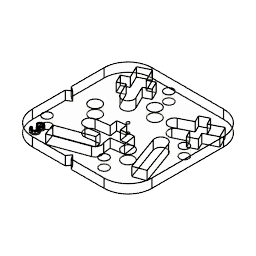
TopPlateTest_v2 (Autodesk Fusion 360 design; units mm, degrees)
Autodesk Fusion 360 part; units mm, degrees
sketch "Sketch1" plane through (0, 0, 0) normal (0, 0, 1) x (1, 0, 0)
  line L0 (55, -55) -> (-55, -55)
  line L1 (-55, -55) -> (-55, 55)
  line L2 (-55, 55) -> (55, 55)
  line L3 (55, 55) -> (55, -55)
  circle A0 centre (0, 9) radius 2
  circle A1 centre (0, -11) radius 1
  circle A2 centre (0, 0) radius 0.5
  circle A3 centre (-27, 47) radius 3
  circle A4 centre (-1, 47) radius 3
  circle A5 centre (46.8686, 27.2241) radius 3
  line L4 (46.9988, 1) -> (46.9855, 27.035) construction
  line L5 (-1, 47) -> (-27, 47) construction
  circle A6 centre (47.0008, 0.9939) radius 3
  circle A7 centre (-47, -1) radius 3
  line L6 (-47.008, -2.9175) -> (-47.0012, -29) construction
  circle A8 centre (-47, -27) radius 3
  circle A9 centre (0.0158, -47.1318) radius 3
  line L7 (1, -47) -> (27, -47) construction
  circle A10 centre (27.9746, -46.6245) radius 3
  line L8 (27.9746, -46.6245) -> (11, 0) construction
  line L9 (0, 0) -> (5, 0) construction
  line L10 (9.1207, -0.6842) -> (12.8793, 0.6842) construction
  line L11 (12.8793, 0.6842) -> (16.9846, -10.5917)
  line L12 (9.1207, -0.6842) -> (13.2259, -11.9602)
  line L13 (16.9846, -10.5917) -> (13.2259, -11.9602)
  circle A11 centre (11, 0) radius 2
  line L14 (-0.6842, -9.1207) -> (-11.9602, -13.2259)
  line L15 (-10.5917, -16.9846) -> (-11.9602, -13.2259)
  line L16 (0.6842, -12.8793) -> (-10.5917, -16.9846)
  circle A12 centre (0, -11) radius 2
  line L17 (-46.6245, -27.9746) -> (0, -11) construction
  circle A13 centre (7.7782, 7.7782) radius 2
  line L18 (7.7782, 7.7782) -> (46.8686, 27.2241) construction
  line L19 (7.7782, 7.7782) -> (8.669, 5.9875) construction
  line L20 (8.669, 5.9875) -> (19.413, 11.3322)
  line L21 (19.413, 11.3322) -> (17.6314, 14.9136)
  line L22 (17.6314, 14.9136) -> (6.8874, 9.5688)
  circle A14 centre (-7.7782, 7.7782) radius 2
  line L23 (-7.7782, 7.7782) -> (-27, 47) construction
  line L24 (-7.7782, 7.7782) -> (-9.5741, 6.898) construction
  line L25 (-9.5741, 6.898) -> (-14.855, 17.6736)
  line L26 (-5.9823, 8.6583) -> (-11.2631, 19.4339)
  line L27 (-11.2631, 19.4339) -> (-14.855, 17.6736)
  line L28 (46.9988, 1) -> (-6.364, -6.364) construction
  line L29 (0.0158, -47.1318) -> (-11, 0) construction
  line L30 (0, 9) -> (-47.008, -2.9175) construction
  circle A15 centre (7.7782, -7.7782) radius 2
  line L31 (7.7782, -7.7782) -> (-1, 47) construction
  line L32 (0, 0) -> (9, 0) construction
  circle A16 centre (-6.364, -6.364) radius 2
  line L33 (0, -11) -> (0.6842, -12.8793)
  circle A17 centre (-11, 0) radius 2
  line L34 (-11, 0) -> (-9.0525, 0.4552) construction
  line L35 (-9.0525, 0.4552) -> (-6.3214, -11.2299)
  line L36 (-6.3214, -11.2299) -> (-10.2164, -12.1403)
  line L37 (-10.2164, -12.1403) -> (-12.9475, -0.4552)
  line L38 (-6.364, -6.364) -> (-6.0906, -8.3452) construction
  line L39 (-6.0906, -8.3452) -> (5.7968, -6.7048)
  line L40 (5.7968, -6.7048) -> (5.25, -2.7423)
  line L41 (5.25, -2.7423) -> (-6.6374, -4.3827)
  line L42 (7.7782, -7.7782) -> (9.753, -7.4617) construction
  line L43 (9.753, -7.4617) -> (7.8542, 4.3871)
  line L44 (7.8542, 4.3871) -> (3.9046, 3.7542)
  line L45 (3.9046, 3.7542) -> (5.8034, -8.0946)
  line L46 (0, 9) -> (0.4915, 7.0613) construction
  line L47 (0.4915, 7.0613) -> (-11.1405, 4.1124)
  line L48 (-11.1405, 4.1124) -> (-12.1235, 7.9897)
  line L49 (-12.1235, 7.9897) -> (-0.4915, 10.9387)
  line L50 (20, -20) -> (-20, -20)
  line L51 (-20, -20) -> (-20, 20)
  line L52 (-20, 20) -> (20, 20)
  line L53 (20, 20) -> (20, -20)
  line L54 (20, -20) -> (-20, 20) construction
  line L55 (-20, -20) -> (20, 20) construction
  line L56 (15.1052, -11.276) -> (11, 0) construction
  line L57 (13.0526, -5.638) -> (14.9319, -4.9538) construction
  line L58 (13.0526, -5.638) -> (11.1733, -6.3222) construction
  line L59 (14.9319, -4.9538) -> (17.2811, -4.0985) construction
  line L60 (16.7679, -2.689) -> (17.7943, -5.508)
  line L61 (17.7943, -5.508) -> (9.3373, -8.5869)
  line L62 (16.7679, -2.689) -> (8.311, -5.7679)
  line L63 (8.311, -5.7679) -> (9.3373, -8.5869)
  line L64 (18.5222, 13.1229) -> (7.7782, 7.7782) construction
  line L65 (13.1502, 10.4505) -> (14.041, 8.6599) construction
  line L66 (14.041, 8.6599) -> (15.1545, 6.4215) construction
  line L67 (13.8115, 5.7534) -> (16.4975, 7.0896)
  line L68 (13.8115, 5.7534) -> (9.8029, 13.8115)
  line L69 (9.8029, 13.8115) -> (12.4889, 15.1476)
  line L70 (12.4889, 15.1476) -> (16.4975, 7.0896)
  line L71 (-13.0591, 18.5537) -> (-7.7782, 7.7782) construction
  line L72 (-10.4186, 13.1659) -> (-6.3778, 15.1463) construction
  line L73 (-7.0379, 16.4932) -> (-5.7177, 13.7993)
  line L74 (-7.0379, 16.4932) -> (-5.7177, 13.7993) construction
  line L75 (-5.7177, 13.7993) -> (-13.7993, 9.8387)
  line L76 (-13.7993, 9.8387) -> (-15.1196, 12.5326)
  line L77 (-15.1196, 12.5326) -> (-7.0379, 16.4932)
  line L78 (0, 9) -> (-11.632, 6.051) construction
  line L79 (-5.816, 7.5255) -> (-4.7101, 3.1635) construction
  line L80 (-6.1642, 2.7949) -> (-3.2561, 3.5321) construction
  line L81 (-3.2561, 3.5321) -> (-6.1642, 2.7949)
  line L82 (-6.1642, 2.7949) -> (-8.3759, 11.5189)
  line L83 (-8.3759, 11.5189) -> (-5.4679, 12.2561)
  line L84 (-5.4679, 12.2561) -> (-3.2561, 3.5321)
  line L85 (-11, 0) -> (-8.2689, -11.6851) construction
  line L86 (-9.6345, -5.8425) -> (-14.0164, -6.8667) construction
  line L87 (-14.3578, -5.4061) -> (-13.675, -8.3273) construction
  line L88 (-14.3578, -5.4061) -> (-13.675, -8.3273)
  line L89 (-13.675, -8.3273) -> (-4.9112, -6.279)
  line L90 (-4.9112, -6.279) -> (-5.5939, -3.3578)
  line L91 (-5.5939, -3.3578) -> (-14.3578, -5.4061)
  line L92 (5.5234, -4.7235) -> (-6.364, -6.364) construction
  line L93 (-0.4203, -5.5437) -> (-1.0354, -1.086) construction
  line L94 (-2.5214, -1.291) -> (0.4505, -0.8809) construction
  line L95 (-2.5214, -1.291) -> (0.4505, -0.8809)
  line L96 (0.4505, -0.8809) -> (1.6808, -9.7965)
  line L97 (1.6808, -9.7965) -> (-1.291, -10.2066)
  line L98 (-1.291, -10.2066) -> (-2.5214, -1.291)
  line L99 (0, -11) -> (-11.276, -15.1052) construction
  line L100 (-5.638, -13.0526) -> (-4.0985, -17.2811) construction
  line L101 (-5.508, -17.7943) -> (-2.689, -16.7679) construction
  line L102 (-2.689, -16.7679) -> (-5.508, -17.7943)
  line L103 (-5.508, -17.7943) -> (-8.5869, -9.3373)
  line L104 (-8.5869, -9.3373) -> (-5.7679, -8.311)
  line L105 (-5.7679, -8.311) -> (-2.689, -16.7679)
  line L106 (7.7782, -7.7782) -> (5.8794, 4.0707) construction
  line L107 (6.8288, -1.8538) -> (11.2721, -1.1417) construction
  line L108 (11.0348, 0.3394) -> (11.5094, -2.6228) construction
  line L109 (11.0348, 0.3394) -> (11.5094, -2.6228)
  line L110 (11.5094, -2.6228) -> (2.6228, -4.0469)
  line L111 (2.6228, -4.0469) -> (2.1481, -1.0847)
  line L112 (2.1481, -1.0847) -> (11.0348, 0.3394)
  line L113 (0, -20) -> (0, -18.5) construction
  line L114 (0, -20) -> (1, -20) construction
  line L115 (0, -20) -> (-1, -20) construction
  line L116 (-1, -20) -> (0, -18.5)
  line L117 (1, -20) -> (0, -18.5)
  line L118 (-20, 0) -> (-18.5, 0) construction
  line L119 (-18.5, 0) -> (-20, 1)
  line L120 (-18.5, 0) -> (-20, -1)
  line L121 (-20, -1) -> (-20, 0) construction
  line L122 (-20, 0) -> (-20, 1) construction
  circle A18 centre (6, -14) radius 1.5
  circle A19 centre (16.1042, 2.7351) radius 1.5
  circle A20 centre (-2.3297, 15.9975) radius 1.5
  circle A21 centre (-15.6755, -11.4449) radius 1.5
  line L123 (-15.2718, -18.2779) -> (-12.2718, -18.2553) construction
  line L124 (-12.2718, -18.2553) -> (-12.3017, -14.291) construction
  line L125 (-12.3017, -14.291) -> (-15.3017, -14.3137) construction
  line L126 (-15.3017, -14.3137) -> (-15.2718, -18.2779) construction
  dimension "d16" = 110
  dimension "d17" = 110
  dimension "d41" = 9
  dimension "d42" = 4
  dimension "d45" = 1
  dimension "d48" = 6
  dimension "d49" = 6
  dimension "d53" = 11
  dimension "d58" = 4
  dimension "d60" = 12
  dimension "d67" = 4
  dimension "d68" = 12
  dimension "d69" = 4
  dimension "d70" = 4
  dimension "d71" = 12
  dimension "d74" = 11
  dimension "d75" = 4
  dimension "d77" = 9
  dimension "d78" = 4
  dimension "d80" = 12
  dimension "d81" = 4
  dimension "d82" = 12
  dimension "d83" = 4
  dimension "d84" = 12
  dimension "d85" = 4
  dimension "d86" = 12
  dimension "d87" = 4
  dimension "d88" = 12
  dimension "d89" = 4
  dimension "d90" = 40
  dimension "d91" = 40
  dimension "d92" = 2.5
  dimension "d93" = 3
  dimension "d94" = 9
  dimension "d95" = 9
  dimension "d96" = 2.5
  dimension "d97" = 3
  dimension "d98" = 9
  dimension "d99" = 3
  dimension "d100" = 4.5
  dimension "d101" = 3
  dimension "d102" = 9
  dimension "d103" = 4.5
  dimension "d104" = 3
  dimension "d105" = 9
  dimension "d106" = 4.5
  dimension "d107" = 3
  dimension "d108" = 9
  dimension "d109" = 4.5
  dimension "d110" = 3
  dimension "d111" = 9
  dimension "d112" = 4.5
  dimension "d113" = 3
  dimension "d114" = 9
  dimension "d115" = 4.5
  dimension "d116" = 3
  dimension "d117" = 9
  dimension "d128" = 1.5
  dimension "d129" = 1
  dimension "d130" = 1
  dimension "d131" = 1.5
  dimension "d132" = 3
  dimension "d133" = 3
  dimension "d134" = 3
  dimension "d135" = 3
  dimension "d136" = 4
  dimension "d137" = 0
  constraint horizontal L0
  constraint perpendicular L0 L1
  constraint parallel L0 L2
  constraint parallel L1 L3
  constraint coincident A2.centre L9.start
  constraint coincident A0.centre L30.start
  constraint coincident A4.centre L5.start
  constraint coincident A3.centre L5.end
  constraint horizontal L5
  constraint coincident A10.centre L8.start
  constraint horizontal L9
  constraint midpoint L8.end L10
  constraint perpendicular L8 L10
  constraint perpendicular L10 L11
  constraint perpendicular L10 L12
  constraint coincident L8.end A11.centre
  constraint coincident L10.start A11
  constraint coincident A5.centre L18.end
  constraint coincident A13 L19.end
  constraint perpendicular L18 L19
  constraint perpendicular L19 L20
  constraint perpendicular L18 L21
  constraint coincident A13 L22.end
  constraint tangent A13 L22
  constraint coincident A14 L24.end
  constraint perpendicular L23 L24
  constraint coincident A14 L26.start
  constraint coincident A9.centre L29.start
  constraint coincident A15.centre L31.start
  constraint horizontal L32
  constraint coincident L28.end A16.centre
  constraint coincident A1.centre A12.centre
  constraint coincident A12 L16.start
  constraint perpendicular L17 L33
  constraint perpendicular L11 L13
  constraint coincident A17 L34.end
  constraint perpendicular L29 L34
  constraint perpendicular L34 L35
  constraint perpendicular L29 L36
  constraint coincident A17 L37.end
  constraint tangent A17 L37
  constraint perpendicular L36 L37
  constraint coincident A16 L38.end
  constraint perpendicular L28 L38
  constraint perpendicular L38 L39
  constraint perpendicular L39 L40
  constraint coincident A16 L41.end
  constraint tangent A16 L41
  constraint coincident A15 L42.end
  constraint perpendicular L31 L42
  constraint perpendicular L42 L43
  constraint perpendicular L43 L44
  constraint coincident A15 L45.end
  constraint tangent A15 L45
  constraint coincident A0 L46.end
  constraint perpendicular L30 L46
  constraint perpendicular L46 L47
  constraint perpendicular L30 L48
  constraint coincident A0 L49.end
  constraint tangent A0 L49
  constraint horizontal L50
  constraint perpendicular L50 L51
  constraint parallel L50 L52
  constraint parallel L51 L53
  constraint coincident L54 A2.centre
  constraint coincident L55 A2.centre
  constraint midpoint L13 L56.start
  constraint midpoint L56 L57.start
  constraint midpoint L11 L57.end
  constraint midpoint L12 L58.end
  constraint perpendicular L11 L59
  constraint midpoint L59.end L60
  constraint perpendicular L59 L60
  constraint perpendicular L12 L61
  constraint perpendicular L12 L62
  constraint midpoint L21 L64.start
  constraint coincident A13.centre L18.start
  constraint perpendicular L19 L64
  constraint midpoint L64 L65.start
  constraint midpoint L20 L65.end
  constraint perpendicular L20 L65
  constraint perpendicular L20 L66
  constraint midpoint L66.end L67
  constraint perpendicular L66 L67
  constraint perpendicular L64 L68
  constraint perpendicular L68 L69
  constraint midpoint L27 L71.start
  constraint coincident A14.centre L23.start
  constraint perpendicular L24 L71
  constraint midpoint L71 L72.start
  constraint perpendicular L26 L72
  constraint midpoint L72.end L73
  constraint perpendicular L72 L73
  constraint perpendicular L74 L75
  constraint parallel L74 L76
  constraint parallel L75 L77
  constraint midpoint L48 L78.end
  constraint midpoint L78 L79.start
  constraint perpendicular L47 L79
  constraint midpoint L79.end L80
  constraint perpendicular L79 L80
  constraint perpendicular L81 L82
  constraint parallel L81 L83
  constraint parallel L82 L84
  constraint coincident L29.end A17.centre
  constraint midpoint L36 L85.end
  constraint midpoint L85 L86.start
  constraint perpendicular L37 L86
  constraint midpoint L86.end L87
  constraint perpendicular L86 L87
  constraint perpendicular L88 L89
  constraint parallel L88 L90
  constraint parallel L89 L91
  constraint midpoint L40 L92.start
  constraint midpoint L92 L93.start
  constraint perpendicular L41 L93
  constraint midpoint L93.end L94
  constraint perpendicular L93 L94
  constraint perpendicular L95 L96
  constraint parallel L95 L97
  constraint parallel L96 L98
  constraint midpoint L15 L99.end
  constraint perpendicular L15 L99
  constraint midpoint L99 L100.start
  constraint perpendicular L16 L100
  constraint midpoint L100.end L101
  constraint perpendicular L100 L101
  constraint perpendicular L102 L103
  constraint parallel L102 L104
  constraint parallel L103 L105
  constraint midpoint L44 L106.end
  constraint midpoint L106 L107.start
  constraint perpendicular L106 L107
  constraint midpoint L107.end L108
  constraint perpendicular L107 L108
  constraint perpendicular L109 L110
  constraint parallel L109 L111
  constraint parallel L110 L112
  constraint midpoint L50 L113.start
  constraint perpendicular L50 L113
  constraint perpendicular L113 L114
  constraint perpendicular L113 L115
  constraint midpoint L51 L118.start
  constraint perpendicular L51 L118
  constraint coincident L51 L119.end
  constraint coincident L51 L120.end
  measures "d16" distance of L1.end L2.end
  measures "d17" distance of L0.end L1.end
  measures "d41" distance of A2.centre A0.centre
  measures "d42" diameter of A0
  measures "d45" diameter of A2
  measures "d48" diameter of A3
  measures "d49" diameter of A4
  measures "d53" distance of A2.centre A13.centre
  measures "d58" distance of L10.start L10.end
  measures "d60" distance of L10.start L12.end
  measures "d67" diameter of A13
  measures "d68" distance of L19.end L20.end
  measures "d69" distance of L20.end L21.end
  measures "d70" diameter of A14
  measures "d71" distance of L24.end L25.end
  measures "d74" distance of A2.centre A15.centre
  measures "d75" diameter of A15
  measures "d77" distance of A2.centre L28.end
  measures "d78" diameter of A16
  measures "d80" distance of L15.start L16.start
  measures "d81" diameter of A17
  measures "d82" distance of L34.end L35.end
  measures "d83" distance of L35.end L36.end
  measures "d84" distance of L38.end L39.end
  measures "d85" distance of L39.end L40.end
  measures "d86" distance of L42.end L43.end
  measures "d87" distance of L43.end L44.end
  measures "d88" distance of L46.end L47.end
  measures "d89" distance of L47.end L48.end
  measures "d90" distance of L51.end L52.end
  measures "d91" distance of L50.end L51.end
  measures "d92" distance of L57.end L59.end
  measures "d93" distance of L60.start L60.end
  measures "d94" distance of L60.end L61.end
  measures "d95" distance of L60.start L62.end
  measures "d96" distance of L65.end L66.end
  measures "d97" distance of L67.start L67.end
  measures "d98" distance of L67.start L68.end
  measures "d99" distance of L68.end L69.end
  measures "d100" distance of L72.start L72.end
  measures "d101" distance of L73.start L73.end
  measures "d102" distance of L73.start L76.end
  measures "d103" distance of L79.start L79.end
  measures "d104" distance of L80.start L80.end
  measures "d105" distance of L80.end L83.end
  measures "d106" distance of L86.start L86.end
  measures "d107" distance of L87.start L87.end
  measures "d108" distance of L87.start L90.end
  measures "d109" distance of L93.start L93.end
  measures "d110" distance of L94.start L94.end
  measures "d111" distance of L94.start L97.end
  measures "d112" distance of L100.start L100.end
  measures "d113" distance of L101.start L101.end
  measures "d114" distance of L101.end L104.end
  measures "d115" distance of L107.start L107.end
  measures "d116" distance of L108.start L108.end
  measures "d117" distance of L108.start L111.end
  measures "d128" distance of L113.start L113.end
  measures "d129" distance of L113.start L114.end
  measures "d130" distance of L113.start L115.end
  measures "d131" distance of L118.start L118.end
  measures "d132" diameter of A18
  measures "d133" diameter of A19
  measures "d134" diameter of A20
  measures "d135" diameter of A21
extrude "Extrude1" add sketch "Sketch1" along normal blind 3 contours L0 L1 L2 L3 | A0 L47 L49 L84 | A14 L26 L47 L49 L82 L84 | L26 L49 L83 L84 | L47 L81 L82 L84 | A14 L26 L49 L82 L83 | A14 L26 L49 | A14 L25 L47 L48 L49 L82 | A14 L25 L26 L49 L75 L82 L83 | L25 L26 L75 L77 | L26 L73 L75 L77 | A14 L25 L49 | L25 L26 L27 L77 | L25 L75 L76 L77 | L14 A12 L39 L96 L97 L98 | L14 L16 A12 L98 L105 | L14 A12 L98 | L16 L102 L103 L105 | L14 L16 L35 L36 L103 L105 | L14 A16 L35 L39 L98 L104 L105 | L39 L41 L45 L96 L110 L111 | L39 L41 L96 L98 | L14 L15 L16 L103 | L14 L35 L104 L105 | A16 L39 L41 L90 L98 | L39 L40 L45 L110 | A15 L39 L40 L43 L45 L62 L63 L110 | L41 L95 L96 L98 | L14 L36 L103 | L14 L35 L36 | L14 L35 L36 L103 L104 | L41 L45 L110 L111 | L40 L41 L45 L110 | L41 L45 L111 L112 | A16 L35 L36 L37 L89 L103 L104 | A16 L41 L90 | A16 L35 L41 L90 L91 | L40 L41 L43 L45 L110 L112 | A15 L43 L62 L63 | L12 A15 L43 L61 L62 | A16 L35 L37 L89 L91 | L12 L43 L62 L110 | L12 A11 L43 L110 L112 | L43 L44 L45 L112 | L11 L12 L13 L61 | L11 L12 L61 L62 | L37 L88 L89 L91 | A17 L35 L37 L91 | L11 L12 A11 L62 L109 L110 | L12 A11 L109 L110 | L11 L60 L61 L62 | A3 | A4 | A5 | A6 | A7 | A8 | A9 | A10 | A13 L20 L22 L68 | L22 L68 L69 L70 | L20 L22 L68 L70 | L20 L67 L68 L70 | L20 L21 L22 L70 | L50 L51 L52 L53 L116 L117 L119 L120
fillet "Fillet1" radius 40 4 edges at (55, -55, 1.5) (-55, -55, 1.5) (55, 55, 1.5) (-55, 55, 1.5)
extrude "Extrude5" cut sketch "Sketch1" along normal blind 3 contours A0 | A14 L26 L49 L82 L83 | A14 L26 L49 | A14 L49 L82 | A14 L25 L26 L49 L75 L82 L83 | A14 L49 L82 | A14 L49 L82 | L25 L26 L75 L77 | L26 L73 L75 L77 | A14 L49 L82 | A14 L25 L49 | L25 L26 L27 L77 | L25 L75 L76 L77 | A1 L97 | A1 A12 L33 L97 | A1 A12 L97 L98 | A1 A12 L33 L97 L98 | L14 A12 L39 L96 L97 L98 | L14 L16 A12 L98 L105 | L14 A12 L98 | L14 L16 L35 L36 L103 L105 | L39 L41 L45 L96 L110 L111 | L39 L41 L96 L98 | L14 L15 L16 L103 | A16 L39 L41 L90 L98 | L41 L95 L96 L98 | L14 L35 L36 | A16 L35 L89 L90 | L41 L45 L110 L111 | A15 L61 L63 | A16 L35 L89 | A16 L41 L90 | A15 L61 L63 | A16 L35 L89 L90 | A16 L35 L89 | L11 L12 L13 L61 | L11 L12 L61 L62 | L11 L12 A11 L62 L109 L110 | L12 A11 L109 L110 | A17 | A11 L109 L112 | A11 L109 L112 | A13 | A13 L20 L22 L68 | L22 L68 L69 L70 | L20 L22 L68 L70 | L20 L67 L68 L70 | L20 L21 L22 L70 picked at (-0.0712, -10.7062)
sketch "Sketch3" plane through (0, 0, 3) normal (0, 0, 1) x (-1, 0, 0)
  circle A0 centre (-6, 14) radius 1.5
  circle A1 centre (15.6755, 11.4449) radius 1.5
  line L0 (-1, 20) -> (1, 20)
  line L1 (1, 20) -> (0, 18.5)
  line L2 (0, 18.5) -> (-1, 20)
  line L3 (-12.8793, -0.6842) -> (-16.9846, 10.5917)
  line L4 (-16.9846, 10.5917) -> (-13.2259, 11.9602)
  line L5 (-13.2259, 11.9602) -> (-9.1207, 0.6842)
  arc A2 (-12.8793, -0.6842) -> (-9.1207, 0.6842) centre (-11, 0) ccw
  circle A3 centre (-16.1042, -2.7351) radius 1.5
  line L6 (20, -1) -> (18.5, 0)
  line L7 (18.5, 0) -> (20, 1)
  line L8 (20, 1) -> (20, -1)
  circle A4 centre (0, -9) radius 2
  circle A5 centre (2.3297, -15.9975) radius 1.5
  circle A6 centre (11, 0) radius 2
  line L9 (-6.8874, -9.5688) -> (-10.9164, -11.5731)
  line L10 (-10.9164, -11.5731) -> (-9.8029, -13.8115)
  line L11 (-9.8029, -13.8115) -> (-12.4889, -15.1476)
  line L12 (-12.4889, -15.1476) -> (-13.6024, -12.9093)
  line L13 (-13.6024, -12.9093) -> (-17.6314, -14.9136)
  line L14 (-17.6314, -14.9136) -> (-19.413, -11.3322)
  line L15 (-19.413, -11.3322) -> (-15.384, -9.328)
  line L16 (-15.384, -9.328) -> (-16.4975, -7.0896)
  line L17 (-16.4975, -7.0896) -> (-13.8115, -5.7534)
  line L18 (-13.8115, -5.7534) -> (-12.698, -7.9918)
  line L19 (-12.698, -7.9918) -> (-8.669, -5.9875)
  arc A7 (-6.8874, -9.5688) -> (-8.669, -5.9875) centre (-7.7782, -7.7782) ccw
  circle A8 centre (-7.7782, 7.7782) radius 2
  circle A9 centre (0, 0) radius 0.5
  arc A10 (15, -55) -> (55, -15) centre (15, -15) ccw
  line L20 (55, -15) -> (55, 15)
  arc A11 (55, 15) -> (15, 55) centre (15, 15) ccw
  line L21 (15, 55) -> (-15, 55)
  arc A12 (-15, 55) -> (-55, 15) centre (-15, 15) ccw
  line L22 (-55, 15) -> (-55, -15)
  arc A13 (-55, -15) -> (-15, -55) centre (-15, -15) ccw
  line L23 (-15, -55) -> (15, -55)
  line L24 (7.9626, -12.6991) -> (5.9823, -8.6583)
  arc A14 (9.5741, -6.898) -> (5.9823, -8.6583) centre (7.7782, -7.7782) ccw
  line L25 (9.5741, -6.898) -> (11.5544, -10.9389)
  line L26 (11.5544, -10.9389) -> (13.7993, -9.8387)
  line L27 (13.7993, -9.8387) -> (15.1196, -12.5326)
  line L28 (15.1196, -12.5326) -> (12.8746, -13.6327)
  line L29 (12.8746, -13.6327) -> (14.855, -17.6736)
  line L30 (14.855, -17.6736) -> (11.2631, -19.4339)
  line L31 (11.2631, -19.4339) -> (9.2828, -15.393)
  line L32 (9.2828, -15.393) -> (7.0379, -16.4932)
  line L33 (7.0379, -16.4932) -> (5.7177, -13.7993)
  line L34 (5.7177, -13.7993) -> (7.9626, -12.6991)
  line L35 (-1.6808, 9.7965) -> (-1.6051, 9.8069)
  arc A15 (-0.6842, 12.8793) -> (-1.6051, 9.8069) centre (0, 11) ccw
  line L36 (-0.6842, 12.8793) -> (10.5917, 16.9846)
  line L37 (10.5917, 16.9846) -> (11.9602, 13.2259)
  line L38 (11.9602, 13.2259) -> (1.4047, 9.383)
  line L39 (1.4047, 9.383) -> (1.6328, 7.73)
  line L40 (1.6328, 7.73) -> (6.0906, 8.3452)
  arc A16 (6.6374, 4.3827) -> (6.0906, 8.3452) centre (6.364, 6.364) ccw
  line L41 (6.6374, 4.3827) -> (2.1796, 3.7676)
  line L42 (2.1796, 3.7676) -> (2.5214, 1.291)
  line L43 (2.5214, 1.291) -> (-0.4505, 0.8809)
  line L44 (-0.4505, 0.8809) -> (-0.7922, 3.3575)
  line L45 (-0.7922, 3.3575) -> (-4.9522, 2.7834)
  line L46 (-4.9522, 2.7834) -> (-5.5853, 6.7339)
  line L47 (-5.5853, 6.7339) -> (-1.339, 7.3199)
  line L48 (-1.339, 7.3199) -> (-1.6808, 9.7965)
  line L49 (15.3036, 18.2575) -> (12.2639, 18.2575) construction
  line L50 (12.2639, 18.2575) -> (12.2639, 14.3136) construction
  line L51 (12.2639, 14.3136) -> (15.3036, 14.3136) construction
  line L52 (15.3036, 14.3136) -> (15.3036, 18.2575) construction
  dimension "d138" = 4
  dimension "d139" = 0
  text T0 "3" font "Arial" height 4 align left top in box 3.0397 x 3.9439 at (15.3036, 18.2575) x (-1, 0) y (0, -1) spacing 1 kerned
extrude "Extrude6" cut sketch "Sketch3" against normal blind 1 text T0
extrude "Extrude7" cut sketch "Sketch1" along normal blind 3 contours L0 L1 L2 L3 | A3 | A4 | A5 | A6 | A7 | A8 | A9 | A10
fillet "Fillet2" radius 8 4 edges at (-20, -20, 1.5) (20, -20, 1.5) (-20, 20, 1.5) (20, 20, 1.5)
equation "d94 = 6.500 mm + 2.5 mm"
equation "d137 = '3'"
equation "d139 = '3'"
